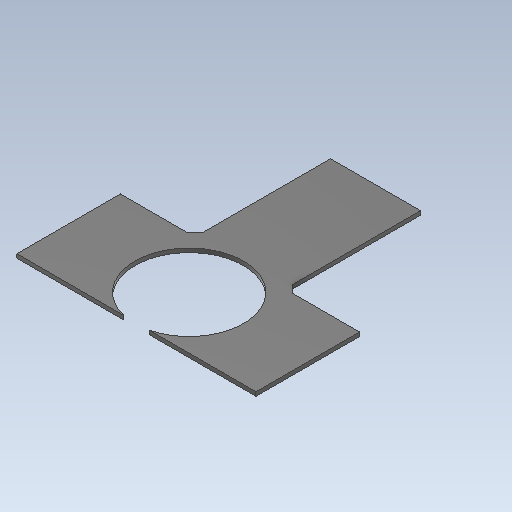
# Autodesk Inventor part: pcb
Saved by Autodesk Inventor 2020 (Build 240168000, 168)
## iProperties
Created: 2020-02-12
Part Number: pcb
Material: UHMW, Black
Document SubType Name: Modeling
Designer: atmat
Density: 0.94 g/cm^3
Appearance: Smooth - Black
Mass: 8.31983 g
Surface Area: 119.197 cm^2
Volume: 8.85088 cm^3
Author: atmat
Autodesk Inventor part; units mm, degrees
ref_plane "YZ Plane" through (0, 0, 0) normal (1, 0, 0) x (0, 1, 0)
ref_plane "XZ Plane" through (0, 0, 0) normal (0, 1, 0) x (-1, 0, 0)
ref_plane "XY Plane" through (0, 0, 0) normal (0, 0, 1) x (1, 0, 0)
sketch "Sketch2" plane through (0, 0, 0) normal (0, 1, 0) x (-1, 0, 0)
  line L0 (48.5, 48.5) -> (-48.5, 48.5)
  line L1 (-48.5, 48.5) -> (-48.5, -48.5)
  line L2 (-48.5, -48.5) -> (48.5, -48.5)
  line L3 (48.5, -48.5) -> (48.5, 48.5)
  circle A0 centre (0, 27.101) radius 22
  line L4 (48.5, -48.5) -> (18.25, -48.5)
  line L5 (18.25, -48.5) -> (18.25, 6.5)
  line L6 (18.25, 6.5) -> (48.5, 6.5)
  line L7 (48.5, 6.5) -> (48.5, -48.5)
  line L8 (-48.5, -48.5) -> (-18.25, -48.5)
  line L9 (-18.25, -48.5) -> (-18.25, 6.5)
  line L10 (-18.25, 6.5) -> (-48.5, 6.5)
  line L11 (-48.5, 6.5) -> (-48.5, -48.5)
  line L12 (21.25, 6.5) -> (18.25, 3.5)
  line L13 (-18.25, 3.5) -> (-21.25, 6.5)
  point P0 (0, 0)
  point P1 (-48.5, 6.5)
  point P2 (18.25, -48.5)
  point P3 (48.5, 6.5)
  dimension "d1" = 44
  dimension "d2" = 97
  dimension "d3" = 97
  dimension "d4" = 48.5
  dimension "d5" = 48.5
  dimension "d7" = 27.101
  dimension "d8" = 30.25
  dimension "d9" = 30.25
  dimension "d10" = 55
  dimension "d11" = 55
  dimension "d14" = 0
  dimension "d15" = 45
  dimension "d16" = 3
  dimension "d17" = 3
  constraints: 28 end point, 6 parallel, 4 perpendicular, 4 point on line, 3 horizontal, 1 centre point
  measures "d1" diameter of A0
  measures "d2" distance of L2.end L0.start
  measures "d3" distance of L0.start L0.end
  measures "d4" distance from line of point (0, 0) L3
  measures "d5" distance from line of L0 point (0, 0)
  measures "d7" distance of point (0, 0) A0.centre
  measures "d8" distance between parallel lines of L1 L9
  measures "d9" distance of L5.end L6.end
  measures "d10" distance between parallel lines of L2 L6
  measures "d11" distance between parallel lines of L2 L10
  measures "d14" horizontal distance of point (0, 0) A0.centre
  measures "d15" angle of L9 L13
  measures "d16" horizontal distance of L12.start L12.end
  measures "d17" horizontal distance of L13.start L13.end
extrude "Extrusion1" add sketch "Sketch2" along normal blind 1.6 contours L3 L6 L5 L2 L9 L10 L1 L0 A0 | L12 L5 L6 | L10 L9 L13
body "Solid1"
